skadis_nut_coupon (Autodesk Fusion 360 design; units mm, degrees)
part number: 2026-09-06-14-40-16-018
Autodesk Fusion 360 part; units mm, degrees
sketch "Plate" plane through (0, 0, 0) normal (0, 1, 0) x (1, 0, 0)
  line L0 (0, 0) -> (11, 0)
  line L1 (11, 0) -> (11, -20)
  line L2 (11, -20) -> (0, -20)
  line L3 (0, -20) -> (0, 0)
  dimension "d174" = 11
  dimension "d175" = 20
  constraint coincident L0.start L3.end
  constraint horizontal L0
  constraint horizontal L2
  constraint vertical L1
  constraint vertical L3
  measures "d174" horizontal distance of L0.start L1.end
  measures "d175" vertical distance of L0.start L1.end
extrude "Plate (1)" add sketch "Plate" along normal mid plane 33 from surface at 4.5
sketch "Screw hole" plane through (0, 0, 0) normal (0, 1, 0) x (1, 0, 0)
  line L0 (-1, -7.6) -> (12, -7.6)
  line L1 (12, -7.6) -> (12, -12.4)
  line L2 (12, -12.4) -> (-1, -12.4)
  line L3 (-1, -12.4) -> (-1, -7.6)
  dimension "d179" = 12
  dimension "d180" = 7.6
  dimension "d181" = 13
  dimension "d182" = 4.8
  constraint horizontal L0
  constraint horizontal L2
  constraint vertical L1
  constraint vertical L3
  measures "d179" horizontal distance of origin L0.end
  measures "d180" vertical distance of origin L0.end
  measures "d181" horizontal distance of L0.start L0.end
  measures "d182" vertical distance of L0.end L1.end
extrude "Screw hole (1)" cut sketch "Screw hole" along normal mid plane 16.8 from surface at 7.52
sketch "Nut cavity" plane through (0, 0, 0) normal (0, 1, 0) x (1, 0, 0)
  line L0 (3.6, -6.3) -> (7, -6.3)
  line L1 (7, -6.3) -> (7, -13.7)
  line L2 (7, -13.7) -> (3.6, -13.7)
  line L3 (3.6, -13.7) -> (3.6, -6.3)
  dimension "d186" = 7
  dimension "d187" = 6.3
  dimension "d188" = 3.4
  dimension "d189" = 7.4
  constraint horizontal L0
  constraint horizontal L2
  constraint vertical L1
  constraint vertical L3
  measures "d186" horizontal distance of origin L0.end
  measures "d187" vertical distance of origin L0.end
  measures "d188" horizontal distance of L0.start L0.end
  measures "d189" vertical distance of L0.end L1.end
extrude "Nut cavity (1)" cut sketch "Nut cavity" along normal mid plane 19.4 from surface at 7.52
sketch "Nut entry" plane through (0, 0, 0) normal (0, 1, 0) x (1, 0, 0)
  line L0 (3.6, -12.7) -> (7, -12.7)
  line L1 (7, -12.7) -> (7, -21)
  line L2 (7, -21) -> (3.6, -21)
  line L3 (3.6, -21) -> (3.6, -12.7)
  dimension "d193" = 7
  dimension "d194" = 12.7
  dimension "d195" = 3.4
  dimension "d196" = 8.3
  constraint horizontal L0
  constraint horizontal L2
  constraint vertical L1
  constraint vertical L3
  measures "d193" horizontal distance of origin L0.end
  measures "d194" vertical distance of origin L0.end
  measures "d195" horizontal distance of L0.start L0.end
  measures "d196" vertical distance of L0.end L1.end
extrude "Nut entry (1)" cut sketch "Nut entry" along normal mid plane 7.4 from surface at 1.52
sketch "Cavity roof" plane through (0, 0, 0) normal (0, 0, 1) x (1, 0, 0)
  line L0 (3.6, -2.18) -> (7, -2.18)
  line L1 (7, -2.18) -> (5.3, -3.88)
  line L2 (5.3, -3.88) -> (3.6, -2.18)
  dimension "d200" = 3.6
  dimension "d201" = 2.18
  dimension "d202" = 7
  dimension "d203" = 5.3
  dimension "d204" = 1.7
  constraint horizontal L0
  measures "d200" horizontal distance of origin L0.start
  measures "d201" vertical distance of origin L0.start
  measures "d202" horizontal distance of origin L0.end
  measures "d203" horizontal distance of origin L1.end
  measures "d204" vertical distance of L0.start L1.end
extrude "Cavity roof (1)" cut sketch "Cavity roof" along normal mid plane 15.7 from surface at 13.15
equation "bracketWidth = 24.0 mm" comment "bracket width across the upright"
equation "plateHeight = 20.0 mm" comment "plate height"
equation "plateInboardExtension = 9.0 mm" comment "extra plate toward the desk centre, where the channel reaches"
equation "boardThickness = 6.0 mm" comment "measured SKADIS panel thickness"
equation "screwLength = 15.0 mm" comment "measured decorative M4 screw"
equation "screwDiameter = 4.0 mm" comment "M4 shank"
equation "screwClearance = 0.8 mm" comment "slack around the shank"
equation "screwTipClearance = 2.0 mm" comment "tip stops this short of the plate's back face"
equation "screwSlotWidth = screwDiameter + screwClearance" comment "screw relief slot height"
equation "nutAcrossFlats = 7.0 mm" comment "M4 square nut across flats"
equation "nutThickness = 3.0 mm" comment "M4 square nut thickness"
equation "nutChannelClearance = 0.4 mm" comment "slack around the nut in its channel"
equation "nutChannelHeight = nutAcrossFlats + nutChannelClearance" comment "channel height; under the nut's diagonal so it cannot turn"
equation "plateThickness = screwLength - boardThickness + screwTipClearance" comment "derived: deep enough to swallow the screw"
equation "mountTravel = 12.0 mm" comment "left-right adjustment"
equation "nutChannelLength = mountTravel + nutAcrossFlats + nutChannelClearance" comment "channel length along the plate"
equation "screwSlotLength = mountTravel + screwSlotWidth" comment "relief slot length along the plate"
equation "topMountZ = 10.0 mm" comment "top channel centre"
equation "mountOffsetY = 7.52 mm" comment "channel centre on the board's grid"
equation "slotOvershoot = 1.0 mm" comment "cuts reach past the faces they cut"
equation "nutCavityClearance = 0.4 mm" comment "slack across the nut's thickness"
equation "nutWallThickness = 4.0 mm" comment "wall in front of the nut; the screw pulls the nut against it"
equation "nutCavityDepth = nutThickness + nutCavityClearance" comment "cavity depth"
equation "nutRoofDepth = nutCavityDepth / 2" comment "45 deg roof beyond the cavity's outboard end, so it prints unsupported"
equation "d174 = plateThickness"
equation "d175 = plateHeight"
equation "d176 = plateInboardExtension / 2"
equation "d177 = bracketWidth + plateInboardExtension"
equation "d179 = plateThickness + slotOvershoot"
equation "d180 = topMountZ - screwSlotWidth / 2"
equation "d181 = plateThickness + 2 * slotOvershoot"
equation "d182 = screwSlotWidth"
equation "d183 = mountOffsetY"
equation "d184 = screwSlotLength"
equation "d186 = plateThickness - nutWallThickness"
equation "d187 = topMountZ - nutChannelHeight / 2"
equation "d188 = nutCavityDepth"
equation "d189 = nutChannelHeight"
equation "d190 = mountOffsetY"
equation "d191 = nutChannelLength"
equation "d193 = plateThickness - nutWallThickness"
equation "d194 = topMountZ + nutChannelHeight / 2 - slotOvershoot"
equation "d195 = nutCavityDepth"
equation "d196 = plateHeight - topMountZ - nutChannelHeight / 2 + 2 * slotOvershoot"
equation "d197 = mountOffsetY - mountTravel / 2"
equation "d198 = nutChannelHeight"
equation "d200 = plateThickness - nutWallThickness - nutCavityDepth"
equation "d201 = -( mountOffsetY - nutChannelLength / 2 )"
equation "d202 = plateThickness - nutWallThickness"
equation "d203 = plateThickness - nutWallThickness - nutCavityDepth / 2"
equation "d204 = nutRoofDepth"
equation "d205 = ( topMountZ - nutChannelHeight / 2 + plateHeight ) / 2"
equation "d206 = plateHeight - topMountZ + nutChannelHeight / 2 + 2 * slotOvershoot"
named bodies: "skadis_nut_coupon"
